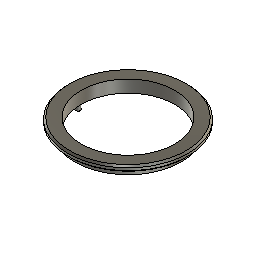
Compact_Robot_MBR1 v1 (Autodesk Fusion 360 design; units mm, degrees)
Autodesk Fusion 360 part; units mm, degrees
sketch "Esboço1" plane through (0, 0, 0) normal (0, 0, 1) x (1, 0, 0)
  circle A0 centre (100, 50) radius 36.5
  circle A1 centre (100, 50) radius 28.5
  dimension "d1" = 73
  dimension "d2" = 57
  constraint concentric A0 A1
  measures "d1" diameter of A0
  measures "d2" diameter of A1
extrude "Extrusão1" add sketch "Esboço1" along normal blind 3.5
sketch "Esboço2" plane through (0, 0, 0) normal (0, 0, -1) x (1, 0, 0)
  circle A0 centre (100, -50) radius 28.5
  circle A1 centre (100, -50) radius 36.5
  circle A2 centre (100, -50) radius 32.5
  dimension "d5" = 65
  constraint concentric A0 A2
  measures "d5" diameter of A2
extrude "Extrusão2" add sketch "Esboço2" along normal blind 4 contours A2
sketch "Esboço3" plane through (0, 0, -4) normal (0, 0, -1) x (1, 0, 0)
  circle A0 centre (100, -50) radius 28.5
  circle A1 centre (100, -50) radius 32.5
  line L0 (55, -50) -> (160, -50) construction
  circle A2 centre (69.4606, -50) radius 1.5
  dimension "d8" = 3
  constraint horizontal L0
  constraint coincident L0 A2.centre
  measures "d8" diameter of A2
extrude "Extrusão3" add sketch "Esboço3" along normal blind 4 contours A2
chamfer "Chanfro1" distance 1 angle 45 2 edges at (65.9701, 36.801, 0) (65.9701, 36.801, 3.5)
chamfer "Chanfro2" distance 0.5 angle 45 1 edges at (68.0621, 50.5424, -8)
